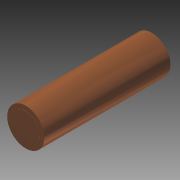
# Autodesk Inventor part: AABattery
Saved by Autodesk Inventor 2012 (Build 160160000, 160)
## iProperties
Created: 2013-12-16
Part Number: AABattery
Material: Default
Document SubType Name: Modeling
Designer: joe_000
Density: 1 g/cm^3
AABatteryDiameter: 14.500 mm
AABatteryLength: 50.500 mm
Author: joe_000
Autodesk Inventor part; units mm, degrees
ref_plane "YZ Plane" through (0, 0, 0) normal (1, 0, 0) x (0, 1, 0)
ref_plane "XZ Plane" through (0, 0, 0) normal (0, 1, 0) x (-1, 0, 0)
ref_plane "XY Plane" through (0, 0, 0) normal (0, 0, 1) x (1, 0, 0)
sketch "Sketch1" plane through (0, 0, 0) normal (0, 1, 0) x (-1, 0, 0)
  circle A0 centre (0, 0) radius 7.25
  dimension "AABatteryDiameter" = 14.5
  constraints: 1 centre point, 1 coincident
  measures "AABatteryDiameter" diameter of A0
extrude "Extrusion1" add sketch "Sketch1" along normal blind 49.4
sketch "Sketch2" plane through (0, 49.4, 0) normal (0, 1, 0) x (1, 0, 0)
  circle A0 centre (0, 0) radius 7.25 projected
  circle A1 centre (0, 0) radius 2.75
  dimension "d3" = 5.5
  constraints: 1 centre point, 1 coincident
  measures "d3" diameter of A1
extrude "Extrusion2" add sketch "Sketch2" along normal blind 1 contours A1
sketch "Sketch3" plane through (0, 0, 0) normal (0, -1, 0) x (1, 0, 0)
  circle A0 centre (0, 0) radius 7.25 projected
  circle A1 centre (0, 0) radius 5.5
  dimension "d6" = 11
  constraints: 1 centre point, 1 coincident
  measures "d6" diameter of A1
extrude "Extrusion3" add sketch "Sketch3" along normal blind 0.1 contours A1
equation "\"AABatteryLength\" = d4 + d1 + d7"
equation "\"d4\" = 1"
equation "\"d1\" = 49.4"
equation "\"d7\" = 0.1"
body "Solid1"
